Autodesk Fusion 360 part; units mm, degrees
(part 4 of 6)
  spline S1122 degree 3 poles (-50.344, 15.3773) (-50.4556, 15.307) (-50.5645, 15.241) (-50.6872, 15.1921) knots 0 0 0 0 1 1 1 1
  spline S1123 degree 3 poles (-50.6872, 15.1921) (-50.6691, 15.2109) (-50.651, 15.2297) (-50.6323, 15.2491) knots 0 0 0 0 1 1 1 1
  spline S1124 degree 3 poles (-50.6323, 15.2491) (-50.4501, 15.4534) (-50.3811, 15.6233) (-50.3221, 15.8884) knots 0 0 0 0 1 1 1 1
  spline S1125 degree 3 poles (-50.3221, 15.8884) (-50.1794, 16.4731) (-49.682, 16.8133) (-49.2179, 17.1446) knots 0 0 0 0 1 1 1 1
  spline S1126 degree 3 poles (-49.2179, 17.1446) (-49.0182, 17.2877) (-48.8217, 17.435) (-48.6251, 17.5823) knots 0 0 0 0 1 1 1 1
  spline S1127 degree 3 poles (-48.6251, 17.5823) (-48.5603, 17.6304) (-48.4948, 17.6776) (-48.4293, 17.7247) knots 0 0 0 0 1 1 1 1
  spline S1128 degree 3 poles (-48.4293, 17.7247) (-48.0216, 18.0274) (-47.557, 18.5172) (-47.4394, 19.0281) knots 0 0 0 0 1 1 1 1
  spline S1129 degree 3 poles (-47.4394, 19.0281) (-47.463, 19.2434) (-47.4932, 19.4392) (-47.6255, 19.6149) knots 0 0 0 0 1 1 1 1
  spline S1130 degree 3 poles (-47.6255, 19.6149) (-48.0279, 19.8024) (-48.4467, 19.7521) (-48.8536, 19.61) knots 0 0 0 0 1 1 1 1
  spline S1131 degree 3 poles (-48.8536, 19.61) (-49.2499, 19.4463) (-49.6121, 19.2138) (-49.9763, 18.9893) knots 0 0 0 0 1 1 1 1
  spline S1132 degree 3 poles (-49.9763, 18.9893) (-50.2765, 18.8143) (-50.6627, 18.7282) (-51.0047, 18.8097) knots 0 0 0 0 1 1 1 1
  spline S1133 degree 3 poles (-51.0047, 18.8097) (-51.0936, 18.8443) (-51.1659, 18.8904) (-51.2454, 18.943) knots 0 0 0 0 1 1 1 1
  spline S1134 degree 3 poles (-51.2454, 18.943) (-51.389, 19.034) (-51.4771, 19.0454) (-51.6426, 19.014) knots 0 0 0 0 1 1 1 1
  spline S1135 degree 3 poles (-51.6426, 19.014) (-51.7259, 18.9745) (-51.7259, 18.9745) (-51.8388, 18.8732) knots 0 0 0 0 1 1 1 1
  spline S1136 degree 3 poles (-51.8388, 18.8732) (-51.9741, 18.7595) (-52.1019, 18.7139) (-52.2735, 18.6677) knots 0 0 0 0 1 1 1 1
  spline S1137 degree 3 poles (-52.2735, 18.6677) (-52.331, 18.6516) (-52.3884, 18.6356) (-52.4459, 18.6195) knots 0 0 0 0 1 1 1 1
  spline S1138 degree 3 poles (-52.4459, 18.6195) (-52.4756, 18.6115) (-52.5054, 18.6034) (-52.536, 18.5951) knots 0 0 0 0 1 1 1 1
  spline S1139 degree 3 poles (-52.536, 18.5951) (-53.1106, 18.439) (-53.6573, 18.2525) (-54.198, 18.0016) knots 0 0 0 0 1 1 1 1
  spline S1140 degree 3 poles (-54.198, 18.0016) (-54.6047, 17.814) (-55.0066, 17.6569) (-55.4376, 17.5352) knots 0 0 0 0 1 1 1 1
  spline S1141 degree 3 poles (-55.4376, 17.5352) (-55.4604, 17.5687) (-55.4604, 17.5687) (-55.4836, 17.6029) knots 0 0 0 0 1 1 1 1
  spline S1142 degree 3 poles (-55.4836, 17.6029) (-55.6209, 17.7753) (-55.8226, 17.8559) (-56.0361, 17.884) knots 0 0 0 0 1 1 1 1
  spline S1143 degree 3 poles (-56.0361, 17.884) (-56.1445, 17.8761) (-56.2456, 17.8642) (-56.3522, 17.8463) knots 0 0 0 0 1 1 1 1
  spline S1144 degree 3 poles (-56.3522, 17.8463) (-56.3919, 17.8414) (-56.3919, 17.8414) (-56.4323, 17.8363) knots 0 0 0 0 1 1 1 1
  spline S1145 degree 3 poles (-56.4323, 17.8363) (-57.0096, 17.7406) (-57.5367, 17.3205) (-58.0104, 16.9992) knots 0 0 0 0 1 1 1 1
  spline S1146 degree 3 poles (-58.0104, 16.9992) (-58.3797, 16.7497) (-58.7477, 16.5551) (-59.1587, 16.3833) knots 0 0 0 0 1 1 1 1
  spline S1147 degree 3 poles (-59.1587, 16.3833) (-59.2277, 16.3521) (-59.2965, 16.3206) (-59.3651, 16.2885) knots 0 0 0 0 1 1 1 1
  spline S1148 degree 3 poles (-59.3651, 16.2885) (-59.3944, 16.275) (-59.4236, 16.2614) (-59.4537, 16.2474) knots 0 0 0 0 1 1 1 1
  spline S1149 degree 3 poles (-59.4537, 16.2474) (-59.5111, 16.2206) (-59.5686, 16.1938) (-59.626, 16.167) knots 0 0 0 0 1 1 1 1
  spline S1150 degree 3 poles (-59.626, 16.167) (-59.6549, 16.1536) (-59.6837, 16.1402) (-59.7135, 16.1264) knots 0 0 0 0 1 1 1 1
  spline S1151 degree 3 poles (-59.7135, 16.1264) (-59.7417, 16.1133) (-59.7699, 16.1002) (-59.7989, 16.0867) knots 0 0 0 0 1 1 1 1
  spline S1152 degree 3 poles (-59.7989, 16.0867) (-59.8853, 16.0485) (-59.9727, 16.015) (-60.0609, 15.9812) knots 0 0 0 0 1 1 1 1
  spline S1153 degree 3 poles (-60.0609, 15.9812) (-60.2413, 15.907) (-60.3774, 15.8013) (-60.5265, 15.6775) knots 0 0 0 0 1 1 1 1
  spline S1154 degree 3 poles (-60.5265, 15.6775) (-60.8228, 15.4401) (-61.1293, 15.22) (-61.4422, 15.0053) knots 0 0 0 0 1 1 1 1
  spline S1155 degree 3 poles (-61.4422, 15.0053) (-61.4931, 14.9704) (-61.544, 14.9352) (-61.5948, 14.9) knots 0 0 0 0 1 1 1 1
  spline S1156 degree 3 poles (-61.5948, 14.9) (-61.667, 14.85) (-61.7395, 14.8004) (-61.8121, 14.751) knots 0 0 0 0 1 1 1 1
  spline S1157 degree 3 poles (-61.8121, 14.751) (-61.8541, 14.7222) (-61.8962, 14.6934) (-61.9395, 14.6637) knots 0 0 0 0 1 1 1 1
  spline S1158 degree 3 poles (-61.9395, 14.6637) (-62.1493, 14.5407) (-62.3244, 14.4856) (-62.5654, 14.5176) knots 0 0 0 0 1 1 1 1
  spline S1159 degree 3 poles (-62.5654, 14.5176) (-63.3565, 14.5876) (-64.0549, 14.3462) (-64.6704, 13.8507) knots 0 0 0 0 1 1 1 1
  spline S1160 degree 3 poles (-64.6704, 13.8507) (-64.9868, 13.5794) (-65.2483, 13.2746) (-65.5102, 12.952) knots 0 0 0 0 1 1 1 1
  spline S1161 degree 3 poles (-65.5102, 12.952) (-65.5405, 12.9147) (-65.5405, 12.9147) (-65.5715, 12.8767) knots 0 0 0 0 1 1 1 1
  spline S1162 degree 3 poles (-65.5715, 12.8767) (-65.6101, 12.8292) (-65.6485, 12.7816) (-65.6867, 12.7337) knots 0 0 0 0 1 1 1 1
  spline S1163 degree 3 poles (-65.6867, 12.7337) (-66.0286, 12.3111) (-66.4249, 11.9667) (-66.8463, 11.6259) knots 0 0 0 0 1 1 1 1
  spline S1164 degree 3 poles (-66.8463, 11.6259) (-67.102, 11.4159) (-67.3243, 11.1965) (-67.5345, 10.941) knots 0 0 0 0 1 1 1 1
  spline S1165 degree 3 poles (-67.5345, 10.941) (-67.5595, 10.9112) (-67.5845, 10.8815) (-67.6103, 10.8508) knots 0 0 0 0 1 1 1 1
  spline S1166 degree 3 poles (-67.6103, 10.8508) (-68.0141, 10.3567) (-68.1173, 9.5556) (-68.0597, 8.9377) knots 0 0 0 0 1 1 1 1
  spline S1167 degree 3 poles (-68.0597, 8.9377) (-67.8934, 7.6051) (-67.2744, 6.568) (-66.5667, 5.4526) knots 0 0 0 0 1 1 1 1
  spline S1168 degree 3 poles (-66.5667, 5.4526) (-66.5415, 5.4125) (-66.5163, 5.3724) (-66.4904, 5.3311) knots 0 0 0 0 1 1 1 1
  spline S1169 degree 3 poles (-66.4904, 5.3311) (-66.4655, 5.2916) (-66.4405, 5.2522) (-66.4148, 5.2115) knots 0 0 0 0 1 1 1 1
  spline S1170 degree 3 poles (-66.4148, 5.2115) (-66.3924, 5.1759) (-66.37, 5.1403) (-66.3468, 5.1036) knots 0 0 0 0 1 1 1 1
  spline S1171 degree 3 poles (-66.3468, 5.1036) (-66.1436, 4.8029) (-65.891, 4.673) (-65.5627, 4.5317) knots 0 0 0 0 1 1 1 1
  spline S1172 degree 3 poles (-65.5627, 4.5317) (-65.4217, 4.4709) (-65.2852, 4.4033) (-65.1485, 4.3335) knots 0 0 0 0 1 1 1 1
  spline S1173 degree 3 poles (-65.1485, 4.3335) (-64.5048, 4.0056) (-63.893, 3.8018) (-63.1622, 3.8179) knots 0 0 0 0 1 1 1 1
  spline S1174 degree 3 poles (-63.1622, 3.8179) (-63.0974, 3.8188) (-63.0974, 3.8188) (-63.0313, 3.8198) knots 0 0 0 0 1 1 1 1
  spline S1175 degree 3 poles (-63.0313, 3.8198) (-62.9408, 3.8211) (-62.8502, 3.8227) (-62.7596, 3.8245) knots 0 0 0 0 1 1 1 1
  spline S1176 degree 3 poles (-62.7596, 3.8245) (-62.622, 3.8272) (-62.4844, 3.8293) (-62.3467, 3.8313) knots 0 0 0 0 1 1 1 1
  spline S1177 degree 3 poles (-62.3467, 3.8313) (-62.2582, 3.8327) (-62.1696, 3.8341) (-62.081, 3.8356) knots 0 0 0 0 1 1 1 1
  spline S1178 degree 3 poles (-62.081, 3.8356) (-62.0201, 3.8366) (-62.0201, 3.8366) (-61.958, 3.8376) knots 0 0 0 0 1 1 1 1
  spline S1179 degree 3 poles (-61.958, 3.8376) (-60.1229, 3.8743) (-58.2945, 4.4626) (-56.8097, 5.5496) knots 0 0 0 0 1 1 1 1
  spline S1180 degree 3 poles (-56.8097, 5.5496) (-56.6794, 5.6468) (-56.6794, 5.6468) (-56.5257, 5.6878) knots 0 0 0 0 1 1 1 1
  spline S1181 degree 3 poles (-56.5257, 5.6878) (-56.439, 5.6747) (-56.439, 5.6747) (-56.3829, 5.6059) knots 0 0 0 0 1 1 1 1
  spline S1182 degree 3 poles (-56.3829, 5.6059) (-56.2885, 5.4409) (-56.2394, 5.2593) (-56.1818, 5.0789) knots 0 0 0 0 1 1 1 1
  spline S1183 degree 3 poles (-56.1818, 5.0789) (-56.1663, 5.031) (-56.1509, 4.983) (-56.1349, 4.9336) knots 0 0 0 0 1 1 1 1
  spline S1184 degree 3 poles (-56.1349, 4.9336) (-55.9815, 4.4497) (-55.8516, 3.9594) (-55.7199, 3.4693) knots 0 0 0 0 1 1 1 1
  spline S1185 degree 3 poles (-55.7199, 3.4693) (-55.1814, 1.4664) (-54.5799, -0.5857) (-52.7021, -1.7273) knots 0 0 0 0 1 1 1 1
  spline S1186 degree 3 poles (-52.7021, -1.7273) (-52.1368, -2.0407) (-52.1368, -2.0407) (-51.9904, -2.0149) knots 0 0 0 0 1 1 1 1
  spline S1187 degree 3 poles (-51.9904, -2.0149) (-51.9906, -2.0524) (-51.9908, -2.0899) (-51.991, -2.1286) knots 0 0 0 0 1 1 1 1
  spline S1188 degree 3 poles (-51.991, -2.1286) (-51.9636, -2.8299) (-51.645, -3.4042) (-51.3097, -4.0015) knots 0 0 0 0 1 1 1 1
  spline S1189 degree 3 poles (-51.3097, -4.0015) (-51.3453, -4.0094) (-51.3453, -4.0094) (-51.3816, -4.0174) knots 0 0 0 0 1 1 1 1
  spline S1190 degree 3 poles (-51.3816, -4.0174) (-52.0739, -4.1867) (-52.7152, -4.5109) (-53.2315, -5.0035) knots 0 0 0 0 1 1 1 1
  spline S1191 degree 3 poles (-53.2315, -5.0035) (-53.3705, -5.1323) (-53.4674, -5.2003) (-53.6593, -5.2006) knots 0 0 0 0 1 1 1 1
  spline S1192 degree 3 poles (-53.6593, -5.2006) (-53.7599, -5.1657) (-53.8483, -5.129) (-53.9434, -5.0829) knots 0 0 0 0 1 1 1 1
  spline S1193 degree 3 poles (-53.9434, -5.0829) (-55.9004, -4.2074) (-58.0187, -5.0468) (-59.9027, -5.7123) knots 0 0 0 0 1 1 1 1
  spline S1194 degree 3 poles (-59.9027, -5.7123) (-60.2035, -5.8184) (-60.5051, -5.9214) (-60.8077, -6.0222) knots 0 0 0 0 1 1 1 1
  spline S1195 degree 3 poles (-60.8077, -6.0222) (-60.8482, -6.0358) (-60.8886, -6.0493) (-60.9303, -6.0633) knots 0 0 0 0 1 1 1 1
  spline S1196 degree 3 poles (-60.9303, -6.0633) (-61.0381, -6.099) (-61.1461, -6.1339) (-61.2544, -6.1681) knots 0 0 0 0 1 1 1 1
  spline S1197 degree 3 poles (-61.2544, -6.1681) (-61.2996, -6.1825) (-61.2996, -6.1825) (-61.3456, -6.1972) knots 0 0 0 0 1 1 1 1
  spline S1198 degree 3 poles (-61.3456, -6.1972) (-61.6363, -6.2846) (-61.934, -6.3369) (-62.2324, -6.3895) knots 0 0 0 0 1 1 1 1
  spline S1199 degree 3 poles (-62.2324, -6.3895) (-62.3222, -6.4054) (-62.4119, -6.422) (-62.5016, -6.4386) knots 0 0 0 0 1 1 1 1
  spline S1200 degree 3 poles (-62.5016, -6.4386) (-63.1944, -6.5706) (-63.1944, -6.5706) (-63.8495, -6.3701) knots 0 0 0 0 1 1 1 1
  spline S1201 degree 3 poles (-63.8495, -6.3701) (-63.8786, -6.3546) (-63.9077, -6.339) (-63.9377, -6.323) knots 0 0 0 0 1 1 1 1
  spline S1202 degree 3 poles (-63.9377, -6.323) (-63.9949, -6.2924) (-64.0519, -6.2614) (-64.1086, -6.2299) knots 0 0 0 0 1 1 1 1
  spline S1203 degree 3 poles (-64.1086, -6.2299) (-64.1998, -6.18) (-64.2933, -6.1357) (-64.3868, -6.0905) knots 0 0 0 0 1 1 1 1
  spline S1204 degree 3 poles (-64.3868, -6.0905) (-64.5845, -5.986) (-64.761, -5.8541) (-64.942, -5.7237) knots 0 0 0 0 1 1 1 1
  spline S1205 degree 3 poles (-64.942, -5.7237) (-65.255, -5.4989) (-65.5487, -5.3398) (-65.9234, -5.2384) knots 0 0 0 0 1 1 1 1
  spline S1206 degree 3 poles (-65.9234, -5.2384) (-66.0477, -5.198) (-66.1425, -5.1475) (-66.2555, -5.0827) knots 0 0 0 0 1 1 1 1
  spline S1207 degree 3 poles (-66.2555, -5.0827) (-67.2908, -4.5046) (-68.5469, -4.3059) (-69.7187, -4.3147) knots 0 0 0 0 1 1 1 1
  spline S1208 degree 3 poles (-69.7187, -4.3147) (-69.7712, -4.3147) (-69.8237, -4.3147) (-69.8778, -4.3147) knots 0 0 0 0 1 1 1 1
  spline S1209 degree 3 poles (-69.8778, -4.3147) (-70.2207, -4.3231) (-70.5539, -4.37) (-70.8918, -4.426) knots 0 0 0 0 1 1 1 1
  spline S1210 degree 3 poles (-70.8918, -4.426) (-70.9339, -4.4327) (-70.9759, -4.4394) (-71.0192, -4.4463) knots 0 0 0 0 1 1 1 1
  spline S1211 degree 3 poles (-71.0192, -4.4463) (-71.5269, -4.5363) (-71.9207, -4.7633) (-72.2275, -5.1851) knots 0 0 0 0 1 1 1 1
  spline S1212 degree 3 poles (-72.2275, -5.1851) (-72.3637, -5.399) (-72.4828, -5.6214) (-72.5986, -5.8468) knots 0 0 0 0 1 1 1 1
  spline S1213 degree 3 poles (-72.5986, -5.8468) (-72.6546, -5.9506) (-72.7163, -6.0487) (-72.7801, -6.1479) knots 0 0 0 0 1 1 1 1
  spline S1214 degree 3 poles (-72.7801, -6.1479) (-72.9035, -6.3449) (-72.9941, -6.549) (-73.0848, -6.7625) knots 0 0 0 0 1 1 1 1
  spline S1215 degree 3 poles (-73.0848, -6.7625) (-73.2634, -7.1723) (-73.4816, -7.563) (-73.7041, -7.9502) knots 0 0 0 0 1 1 1 1
  spline S1216 degree 3 poles (-73.7041, -7.9502) (-73.7179, -7.9743) (-73.7316, -7.9983) (-73.7458, -8.023) knots 0 0 0 0 1 1 1 1
  spline S1217 degree 3 poles (-73.7458, -8.023) (-73.9174, -8.3215) (-74.0931, -8.6166) (-74.2768, -8.9079) knots 0 0 0 0 1 1 1 1
  spline S1218 degree 3 poles (-74.2768, -8.9079) (-74.3558, -9.0336) (-74.4324, -9.1607) (-74.5089, -9.288) knots 0 0 0 0 1 1 1 1
  spline S1219 degree 3 poles (-74.5089, -9.288) (-74.5741, -9.3949) (-74.6411, -9.5007) (-74.708, -9.6066) knots 0 0 0 0 1 1 1 1
  spline S1220 degree 3 poles (-74.708, -9.6066) (-74.8384, -9.8136) (-74.9561, -10.0259) (-75.0703, -10.2421) knots 0 0 0 0 1 1 1 1
  spline S1221 degree 3 poles (-75.0703, -10.2421) (-75.143, -10.3569) (-75.2065, -10.4303) (-75.3186, -10.5068) knots 0 0 0 0 1 1 1 1
  spline S1222 degree 3 poles (-75.3186, -10.5068) (-75.4881, -10.5374) (-75.6201, -10.4209) (-75.755, -10.3308) knots 0 0 0 0 1 1 1 1
  spline S1223 degree 3 poles (-75.755, -10.3308) (-75.7812, -10.3136) (-75.8075, -10.2965) (-75.8345, -10.2788) knots 0 0 0 0 1 1 1 1
  spline S1224 degree 3 poles (-75.8345, -10.2788) (-76.0434, -10.1412) (-76.2473, -9.9967) (-76.4513, -9.852) knots 0 0 0 0 1 1 1 1
  spline S1225 degree 3 poles (-76.4513, -9.852) (-76.7266, -9.6571) (-77.0027, -9.4835) (-77.3026, -9.3283) knots 0 0 0 0 1 1 1 1
  spline S1226 degree 3 poles (-77.3026, -9.3283) (-77.3412, -9.3073) (-77.3798, -9.2863) (-77.4196, -9.2647) knots 0 0 0 0 1 1 1 1
  spline S1227 degree 3 poles (-77.4196, -9.2647) (-78.1033, -8.9074) (-78.9925, -8.6536) (-79.7502, -8.8776) knots 0 0 0 0 1 1 1 1
  spline S1228 degree 3 poles (-79.7502, -8.8776) (-79.9183, -8.9311) (-80.083, -8.9914) (-80.2475, -9.055) knots 0 0 0 0 1 1 1 1
  spline S1229 degree 3 poles (-80.2475, -9.055) (-80.2801, -9.067) (-80.3128, -9.0791) (-80.3464, -9.0915) knots 0 0 0 0 1 1 1 1
  spline S1230 degree 3 poles (-80.3464, -9.0915) (-80.6659, -9.2148) (-80.9042, -9.3674) (-81.0849, -9.6647) knots 0 0 0 0 1 1 1 1
  spline S1231 degree 3 poles (-81.0849, -9.6647) (-81.1051, -9.6964) (-81.1254, -9.7281) (-81.1462, -9.7608) knots 0 0 0 0 1 1 1 1
  spline S1232 degree 3 poles (-81.1462, -9.7608) (-81.231, -9.9376) (-81.2647, -10.1121) (-81.3, -10.3042) knots 0 0 0 0 1 1 1 1
  spline S1233 degree 3 poles (-81.3, -10.3042) (-81.3073, -10.3437) (-81.3147, -10.3831) (-81.3223, -10.4238) knots 0 0 0 0 1 1 1 1
  spline S1234 degree 3 poles (-81.3223, -10.4238) (-81.5295, -11.5933) (-81.5096, -12.9952) (-80.9381, -14.071) knots 0 0 0 0 1 1 1 1
  spline S1235 degree 3 poles (-80.9381, -14.071) (-80.8732, -14.1963) (-80.8303, -14.2822) (-80.8599, -14.4236) knots 0 0 0 0 1 1 1 1
  spline S1236 degree 3 poles (-80.8599, -14.4236) (-80.9019, -14.5264) (-80.9506, -14.6213) (-81.0044, -14.7184) knots 0 0 0 0 1 1 1 1
  spline S1237 degree 3 poles (-81.0044, -14.7184) (-81.0227, -14.7536) (-81.041, -14.7887) (-81.0598, -14.825) knots 0 0 0 0 1 1 1 1
  spline S1238 degree 3 poles (-81.0598, -14.825) (-81.2073, -15.1051) (-81.3656, -15.3796) (-81.5308, -15.6497) knots 0 0 0 0 1 1 1 1
  spline S1239 degree 3 poles (-81.5308, -15.6497) (-81.5519, -15.6844) (-81.5519, -15.6844) (-81.5734, -15.7199) knots 0 0 0 0 1 1 1 1
  spline S1240 degree 3 poles (-81.5734, -15.7199) (-81.6024, -15.7672) (-81.6322, -15.8141) (-81.6626, -15.8605) knots 0 0 0 0 1 1 1 1
  spline S1241 degree 3 poles (-81.6626, -15.8605) (-81.818, -16.1078) (-81.7716, -16.2778) (-81.6891, -16.5457) knots 0 0 0 0 1 1 1 1
  spline S1242 degree 3 poles (-80.843, -15.9266) (-80.8068, -15.8705) (-80.771, -15.8142) (-80.7353, -15.7577) knots 0 0 0 0 1 1 1 1
  spline S1243 degree 3 poles (-80.7353, -15.7577) (-80.7071, -15.7131) (-80.7071, -15.7131) (-80.6784, -15.6676) knots 0 0 0 0 1 1 1 1
  spline S1244 degree 3 poles (-80.6784, -15.6676) (-80.5785, -15.5008) (-80.4954, -15.3263) (-80.4118, -15.1509) knots 0 0 0 0 1 1 1 1
  spline S1245 degree 3 poles (-80.4118, -15.1509) (-80.3882, -15.1016) (-80.3882, -15.1016) (-80.364, -15.0514) knots 0 0 0 0 1 1 1 1
  spline S1246 degree 3 poles (-80.364, -15.0514) (-80.3179, -14.9544) (-80.2728, -14.8571) (-80.2278, -14.7596) knots 0 0 0 0 1 1 1 1
  spline S1247 degree 3 poles (-80.2278, -14.7596) (-80.2108, -14.7238) (-80.1938, -14.6879) (-80.1762, -14.651) knots 0 0 0 0 1 1 1 1
  spline S1248 degree 3 poles (-80.1762, -14.651) (-80.1598, -14.6154) (-80.1433, -14.5799) (-80.1264, -14.5433) knots 0 0 0 0 1 1 1 1
  spline S1249 degree 3 poles (-80.1264, -14.5433) (-80.1114, -14.5112) (-80.0963, -14.4791) (-80.0809, -14.446) knots 0 0 0 0 1 1 1 1
  spline S1250 degree 3 poles (-80.0809, -14.446) (-80.0301, -14.294) (-80.0815, -14.1798) (-80.1476, -14.0433) knots 0 0 0 0 1 1 1 1
  spline S1251 degree 3 poles (-80.1476, -14.0433) (-80.6954, -12.8464) (-80.8903, -11.5151) (-80.5312, -10.228) knots 0 0 0 0 1 1 1 1
  spline S1252 degree 3 poles (-80.5312, -10.228) (-80.4467, -10.0048) (-80.3701, -9.8918) (-80.1541, -9.7898) knots 0 0 0 0 1 1 1 1
  spline S1253 degree 3 poles (-80.1541, -9.7898) (-79.4267, -9.4766) (-78.8032, -9.5039) (-78.0723, -9.7688) knots 0 0 0 0 1 1 1 1
  spline S1254 degree 3 poles (-78.0723, -9.7688) (-77.8734, -9.8526) (-77.6883, -9.9555) (-77.5031, -10.0659) knots 0 0 0 0 1 1 1 1
  spline S1255 degree 3 poles (-77.5031, -10.0659) (-77.4672, -10.0871) (-77.4314, -10.1083) (-77.3944, -10.1301) knots 0 0 0 0 1 1 1 1
  spline S1256 degree 3 poles (-77.3944, -10.1301) (-77.1271, -10.2928) (-76.8721, -10.4714) (-76.6168, -10.6519) knots 0 0 0 0 1 1 1 1
  spline S1257 degree 3 poles (-76.6168, -10.6519) (-76.4456, -10.7725) (-76.2734, -10.8881) (-76.0921, -10.9932) knots 0 0 0 0 1 1 1 1
  spline S1258 degree 3 poles (-76.0921, -10.9932) (-76.0312, -11.0288) (-75.9713, -11.0661) (-75.9121, -11.1044) knots 0 0 0 0 1 1 1 1
  spline S1259 degree 3 poles (-75.9121, -11.1044) (-75.8797, -11.1252) (-75.8474, -11.1459) (-75.814, -11.1673) knots 0 0 0 0 1 1 1 1
  spline S1260 degree 3 poles (-75.814, -11.1673) (-75.7711, -11.1954) (-75.7711, -11.1954) (-75.7274, -11.224) knots 0 0 0 0 1 1 1 1
  spline S1261 degree 3 poles (-75.7274, -11.224) (-75.5278, -11.3181) (-75.2741, -11.2787) (-75.0713, -11.2067) knots 0 0 0 0 1 1 1 1
  spline S1262 degree 3 poles (-75.0713, -11.2067) (-74.7292, -11.0157) (-74.5238, -10.8159) (-74.3492, -10.464) knots 0 0 0 0 1 1 1 1
  spline S1263 degree 3 poles (-74.3492, -10.464) (-74.264, -10.2977) (-74.1651, -10.1443) (-74.0624, -9.9884) knots 0 0 0 0 1 1 1 1
  spline S1264 degree 3 poles (-74.0624, -9.9884) (-74.0257, -9.9323) (-73.9891, -9.8762) (-73.9525, -9.8201) knots 0 0 0 0 1 1 1 1
  spline S1265 degree 3 poles (-73.9525, -9.8201) (-73.9355, -9.794) (-73.9185, -9.768) (-73.9009, -9.7411) knots 0 0 0 0 1 1 1 1
  spline S1266 degree 3 poles (-73.9009, -9.7411) (-73.8072, -9.5965) (-73.7188, -9.4489) (-73.6312, -9.3005) knots 0 0 0 0 1 1 1 1
  spline S1267 degree 3 poles (-73.6312, -9.3005) (-73.6026, -9.2523) (-73.5739, -9.204) (-73.5452, -9.1558) knots 0 0 0 0 1 1 1 1
  spline S1268 degree 3 poles (-73.5452, -9.1558) (-73.4792, -9.0446) (-73.4135, -8.9333) (-73.3479, -8.8218) knots 0 0 0 0 1 1 1 1
  spline S1269 degree 3 poles (-73.3479, -8.8218) (-73.2869, -8.7183) (-73.2255, -8.615) (-73.1634, -8.5121) knots 0 0 0 0 1 1 1 1
  spline S1270 degree 3 poles (-73.1634, -8.5121) (-72.8339, -7.9621) (-72.5505, -7.3864) (-72.2794, -6.8058) knots 0 0 0 0 1 1 1 1
  spline S1271 degree 3 poles (-72.2794, -6.8058) (-72.1743, -6.5811) (-72.0542, -6.3717) (-71.9187, -6.1639) knots 0 0 0 0 1 1 1 1
  spline S1272 degree 3 poles (-71.9187, -6.1639) (-71.8471, -6.0501) (-71.7853, -5.9338) (-71.7236, -5.8145) knots 0 0 0 0 1 1 1 1
  spline S1273 degree 3 poles (-71.7236, -5.8145) (-71.5966, -5.5778) (-71.4479, -5.3681) (-71.2082, -5.2383) knots 0 0 0 0 1 1 1 1
  spline S1274 degree 3 poles (-71.2082, -5.2383) (-70.3477, -5.0083) (-69.4148, -4.9839) (-68.5406, -5.1397) knots 0 0 0 0 1 1 1 1
  spline S1275 degree 3 poles (-68.5406, -5.1397) (-68.4876, -5.1476) (-68.4346, -5.1555) (-68.38, -5.1636) knots 0 0 0 0 1 1 1 1
  spline S1276 degree 3 poles (-68.38, -5.1636) (-67.7323, -5.2648) (-67.0898, -5.4522) (-66.5208, -5.7808) knots 0 0 0 0 1 1 1 1
  spline S1277 degree 3 poles (-66.5208, -5.7808) (-66.3054, -5.9041) (-66.0916, -5.9751) (-65.8541, -6.0481) knots 0 0 0 0 1 1 1 1
  spline S1278 degree 3 poles (-65.8541, -6.0481) (-65.6176, -6.127) (-65.439, -6.2519) (-65.2495, -6.4104) knots 0 0 0 0 1 1 1 1
  spline S1279 degree 3 poles (-65.2495, -6.4104) (-64.9135, -6.6853) (-64.5171, -6.862) (-64.1258, -7.0436) knots 0 0 0 0 1 1 1 1
  spline S1280 degree 3 poles (-64.1258, -7.0436) (-64.0896, -7.0607) (-64.0533, -7.0777) (-64.016, -7.0953) knots 0 0 0 0 1 1 1 1
  spline S1281 degree 3 poles (-64.016, -7.0953) (-63.8126, -7.1878) (-63.6441, -7.2436) (-63.4178, -7.2518) knots 0 0 0 0 1 1 1 1
  spline S1282 degree 3 poles (-63.4178, -7.2518) (-63.3923, -7.2548) (-63.3668, -7.2577) (-63.3405, -7.2608) knots 0 0 0 0 1 1 1 1
  spline S1283 degree 3 poles (-63.3405, -7.2608) (-63.0389, -7.2899) (-62.7461, -7.2269) (-62.4507, -7.1724) knots 0 0 0 0 1 1 1 1
  spline S1284 degree 3 poles (-62.4507, -7.1724) (-62.3595, -7.1555) (-62.2682, -7.1393) (-62.1769, -7.1233) knots 0 0 0 0 1 1 1 1
  spline S1285 degree 3 poles (-62.1769, -7.1233) (-61.4499, -6.9935) (-60.7697, -6.7941) (-60.075, -6.5462) knots 0 0 0 0 1 1 1 1
  spline S1286 degree 3 poles (-60.075, -6.5462) (-59.9895, -6.516) (-59.904, -6.4858) (-59.8185, -6.4556) knots 0 0 0 0 1 1 1 1
  spline S1287 degree 3 poles (-59.8185, -6.4556) (-59.6525, -6.397) (-59.4865, -6.3383) (-59.3206, -6.2794) knots 0 0 0 0 1 1 1 1
  spline S1288 degree 3 poles (-59.3206, -6.2794) (-58.9237, -6.1386) (-58.5263, -5.9994) (-58.1273, -5.8646) knots 0 0 0 0 1 1 1 1
  spline S1289 degree 3 poles (-58.1273, -5.8646) (-58.099, -5.8548) (-58.0707, -5.845) (-58.0416, -5.8349) knots 0 0 0 0 1 1 1 1
  spline S1290 degree 3 poles (-58.0416, -5.8349) (-57.2581, -5.5668) (-56.3383, -5.3727) (-55.5083, -5.4466) knots 0 0 0 0 1 1 1 1
  spline S1291 degree 3 poles (-55.5083, -5.4466) (-55.4746, -5.4496) (-55.441, -5.4525) (-55.4063, -5.4555) knots 0 0 0 0 1 1 1 1
  spline S1292 degree 3 poles (-55.4063, -5.4555) (-54.9068, -5.5065) (-54.4283, -5.6469) (-53.9729, -5.8571) knots 0 0 0 0 1 1 1 1
  spline S1293 degree 3 poles (-53.9729, -5.8571) (-53.7028, -5.9614) (-53.4421, -5.9531) (-53.1716, -5.8582) knots 0 0 0 0 1 1 1 1
  spline S1294 degree 3 poles (-53.1716, -5.8582) (-52.9314, -5.7114) (-52.7176, -5.5362) (-52.5139, -5.342) knots 0 0 0 0 1 1 1 1
  spline S1295 degree 3 poles (-52.5139, -5.342) (-52.1859, -5.039) (-51.7321, -4.8925) (-51.3214, -4.735) knots 0 0 0 0 1 1 1 1
  spline S1296 degree 3 poles (-51.3214, -4.735) (-51.2295, -4.6997) (-51.1378, -4.6639) (-51.0462, -4.6281) knots 0 0 0 0 1 1 1 1
  spline S1297 degree 3 poles (-51.0462, -4.6281) (-50.9872, -4.6052) (-50.9283, -4.5824) (-50.8694, -4.5596) knots 0 0 0 0 1 1 1 1
  spline S1298 degree 3 poles (-50.8694, -4.5596) (-50.8422, -4.549) (-50.8151, -4.5384) (-50.7871, -4.5275) knots 0 0 0 0 1 1 1 1
  spline S1299 degree 3 poles (-50.7871, -4.5275) (-50.6485, -4.4746) (-50.5167, -4.4335) (-50.3695, -4.414) knots 0 0 0 0 1 1 1 1
  spline S1300 degree 3 poles (-50.3695, -4.414) (-50.4824, -4.0391) (-50.6371, -3.7061) (-50.8258, -3.3637) knots 0 0 0 0 1 1 1 1
  spline S1301 degree 3 poles (-50.8258, -3.3637) (-50.8757, -3.2724) (-50.9254, -3.1811) (-50.975, -3.0896) knots 0 0 0 0 1 1 1 1
  spline S1302 degree 3 poles (-50.975, -3.0896) (-50.9968, -3.0499) (-51.0186, -3.0102) (-51.0411, -2.9693) knots 0 0 0 0 1 1 1 1
  spline S1303 degree 3 poles (-51.0411, -2.9693) (-51.1903, -2.664) (-51.2838, -2.3242) (-51.2366, -1.9852) knots 0 0 0 0 1 1 1 1
  spline S1304 degree 3 poles (-51.2366, -1.9852) (-51.2267, -1.8226) (-51.2649, -1.7413) (-51.3643, -1.6127) knots 0 0 0 0 1 1 1 1
  spline S1305 degree 3 poles (-51.3643, -1.6127) (-51.5348, -1.4371) (-51.7203, -1.3576) (-51.9451, -1.268) knots 0 0 0 0 1 1 1 1
  spline S1306 degree 3 poles (-51.9451, -1.268) (-52.877, -0.8772) (-53.5414, -0.1547) (-54.0025, 0.7284) knots 0 0 0 0 1 1 1 1
  spline S1307 degree 3 poles (-54.0025, 0.7284) (-54.0163, 0.7548) (-54.0301, 0.7812) (-54.0443, 0.8084) knots 0 0 0 0 1 1 1 1
  spline S1308 degree 3 poles (-54.0443, 0.8084) (-54.2299, 1.1713) (-54.3741, 1.5452) (-54.5022, 1.9317) knots 0 0 0 0 1 1 1 1
  spline S1309 degree 3 poles (-54.5022, 1.9317) (-54.5173, 1.9773) (-54.5325, 2.0228) (-54.548, 2.0697) knots 0 0 0 0 1 1 1 1
  spline S1310 degree 3 poles (-54.548, 2.0697) (-54.7227, 2.6035) (-54.8713, 3.1443) (-55.0197, 3.6858) knots 0 0 0 0 1 1 1 1
  spline S1311 degree 3 poles (-55.0197, 3.6858) (-55.1844, 4.2866) (-55.3525, 4.8853) (-55.5448, 5.478) knots 0 0 0 0 1 1 1 1
  spline S1312 degree 3 poles (-55.5448, 5.478) (-55.5596, 5.524) (-55.5744, 5.57) (-55.5897, 5.6174) knots 0 0 0 0 1 1 1 1
  spline S1313 degree 3 poles (-55.5897, 5.6174) (-55.6108, 5.6814) (-55.6108, 5.6814) (-55.6323, 5.7466) knots 0 0 0 0 1 1 1 1
  spline S1314 degree 3 poles (-55.6323, 5.7466) (-55.6446, 5.7839) (-55.6569, 5.8212) (-55.6695, 5.8597) knots 0 0 0 0 1 1 1 1
  spline S1315 degree 3 poles (-55.6695, 5.8597) (-55.7361, 6.0276) (-55.809, 6.152) (-55.9619, 6.2503) knots 0 0 0 0 1 1 1 1
  spline S1316 degree 3 poles (-55.9619, 6.2503) (-55.9879, 6.267) (-56.0138, 6.2837) (-56.0406, 6.301) knots 0 0 0 0 1 1 1 1
  spline S1317 degree 3 poles (-56.0406, 6.301) (-56.0676, 6.3178) (-56.0945, 6.3346) (-56.1223, 6.3519) knots 0 0 0 0 1 1 1 1
  spline S1318 degree 3 poles (-56.1223, 6.3519) (-56.1621, 6.3779) (-56.1621, 6.3779) (-56.2028, 6.4044) knots 0 0 0 0 1 1 1 1
  spline S1319 degree 3 poles (-56.2028, 6.4044) (-56.3492, 6.4973) (-56.469, 6.5672) (-56.6457, 6.5823) knots 0 0 0 0 1 1 1 1
  spline S1320 degree 3 poles (-56.6457, 6.5823) (-56.7423, 6.5337) (-56.7423, 6.5337) (-56.8407, 6.4577) knots 0 0 0 0 1 1 1 1
  spline S1321 degree 3 poles (-56.8407, 6.4577) (-56.8775, 6.4301) (-56.9143, 6.4024) (-56.9523, 6.3739) knots 0 0 0 0 1 1 1 1
  spline S1322 degree 3 poles (-56.9523, 6.3739) (-56.9913, 6.3438) (-57.0303, 6.3138) (-57.0705, 6.2828) knots 0 0 0 0 1 1 1 1
  spline S1323 degree 3 poles (-57.0705, 6.2828) (-57.4699, 5.9861) (-57.871, 5.7285) (-58.3142, 5.5032) knots 0 0 0 0 1 1 1 1
  spline S1324 degree 3 poles (-58.3142, 5.5032) (-58.3475, 5.4862) (-58.3807, 5.4692) (-58.4149, 5.4516) knots 0 0 0 0 1 1 1 1
  spline S1325 degree 3 poles (-58.4149, 5.4516) (-59.858, 4.7202) (-61.3405, 4.5436) (-62.939, 4.5496) knots 0 0 0 0 1 1 1 1
  spline S1326 degree 3 poles (-62.939, 4.5496) (-63.0584, 4.5495) (-63.1777, 4.5469) (-63.297, 4.5446) knots 0 0 0 0 1 1 1 1
  spline S1327 degree 3 poles (-63.297, 4.5446) (-63.7747, 4.5401) (-64.1846, 4.6787) (-64.6085, 4.8891) knots 0 0 0 0 1 1 1 1
  spline S1328 degree 3 poles (-64.6085, 4.8891) (-64.6377, 4.9035) (-64.6669, 4.918) (-64.6969, 4.9329) knots 0 0 0 0 1 1 1 1
  spline S1329 degree 3 poles (-64.6969, 4.9329) (-64.8806, 5.0244) (-65.0638, 5.1169) (-65.2456, 5.212) knots 0 0 0 0 1 1 1 1
  spline S1330 degree 3 poles (-65.2456, 5.212) (-65.3066, 5.2428) (-65.3685, 5.272) (-65.431, 5.2997) knots 0 0 0 0 1 1 1 1
  spline S1331 degree 3 poles (-65.431, 5.2997) (-65.65, 5.3995) (-65.7528, 5.4853) (-65.8677, 5.7049) knots 0 0 0 0 1 1 1 1
  spline S1332 degree 3 poles (-65.8677, 5.7049) (-65.897, 5.7588) (-65.9264, 5.8127) (-65.9559, 5.8665) knots 0 0 0 0 1 1 1 1
  spline S1333 degree 3 poles (-65.9559, 5.8665) (-65.9711, 5.8948) (-65.9863, 5.923) (-66.002, 5.9522) knots 0 0 0 0 1 1 1 1
  spline S1334 degree 3 poles (-66.002, 5.9522) (-66.0685, 6.0715) (-66.1416, 6.1862) (-66.215, 6.3014) knots 0 0 0 0 1 1 1 1
  spline S1335 degree 3 poles (-66.215, 6.3014) (-66.4131, 6.6128) (-66.5985, 6.9302) (-66.7759, 7.2538) knots 0 0 0 0 1 1 1 1
  spline S1336 degree 3 poles (-66.7759, 7.2538) (-66.7961, 7.2902) (-66.8163, 7.3265) (-66.8371, 7.364) knots 0 0 0 0 1 1 1 1
  spline S1337 degree 3 poles (-66.8371, 7.364) (-67.2901, 8.2014) (-67.4687, 9.1631) (-67.2022, 10.0832) knots 0 0 0 0 1 1 1 1
  spline S1338 degree 3 poles (-67.2022, 10.0832) (-66.9956, 10.6318) (-66.4475, 10.9921) (-66.0162, 11.3556) knots 0 0 0 0 1 1 1 1
  spline S1339 degree 3 poles (-66.0162, 11.3556) (-65.6401, 11.674) (-65.3148, 12.0154) (-65.0181, 12.4096) knots 0 0 0 0 1 1 1 1
  spline S1340 degree 3 poles (-65.0181, 12.4096) (-64.5632, 13.0027) (-64.0203, 13.6014) (-63.2562, 13.7349) knots 0 0 0 0 1 1 1 1
  spline S1341 degree 3 poles (-63.2562, 13.7349) (-63.2209, 13.7411) (-63.1857, 13.7474) (-63.1493, 13.7538) knots 0 0 0 0 1 1 1 1
  spline S1342 degree 3 poles (-63.1493, 13.7538) (-62.8338, 13.804) (-62.5593, 13.7819) (-62.2437, 13.7327) knots 0 0 0 0 1 1 1 1
  spline S1343 degree 3 poles (-62.2437, 13.7327) (-62.0559, 13.7096) (-61.9695, 13.7559) (-61.8157, 13.8629) knots 0 0 0 0 1 1 1 1
  spline S1344 degree 3 poles (-61.8157, 13.8629) (-61.773, 13.8923) (-61.7302, 13.9216) (-61.6862, 13.9519) knots 0 0 0 0 1 1 1 1
  spline S1345 degree 3 poles (-61.6862, 13.9519) (-61.6402, 13.9842) (-61.5942, 14.0166) (-61.5482, 14.049) knots 0 0 0 0 1 1 1 1
  spline S1346 degree 3 poles (-61.5482, 14.049) (-61.5008, 14.0818) (-61.4533, 14.1147) (-61.4059, 14.1475) knots 0 0 0 0 1 1 1 1
  spline S1347 degree 3 poles (-61.4059, 14.1475) (-61.3079, 14.2152) (-61.2102, 14.2833) (-61.1126, 14.3515) knots 0 0 0 0 1 1 1 1
  spline S1348 degree 3 poles (-61.1126, 14.3515) (-60.972, 14.4498) (-60.8308, 14.5472) (-60.6894, 14.6443) knots 0 0 0 0 1 1 1 1
  spline S1349 degree 3 poles (-60.6894, 14.6443) (-60.6037, 14.7033) (-60.518, 14.7624) (-60.4323, 14.8214) knots 0 0 0 0 1 1 1 1
  spline S1350 degree 3 poles (-60.4323, 14.8214) (-60.3924, 14.849) (-60.3524, 14.8765) (-60.3113, 14.9049) knots 0 0 0 0 1 1 1 1
  spline S1351 degree 3 poles (-60.3113, 14.9049) (-60.2742, 14.9306) (-60.237, 14.9564) (-60.1988, 14.983) knots 0 0 0 0 1 1 1 1
  spline S1352 degree 3 poles (-60.1988, 14.983) (-60.1664, 15.0054) (-60.1341, 15.0278) (-60.1008, 15.0509) knots 0 0 0 0 1 1 1 1
  spline S1353 degree 3 poles (-60.1008, 15.0509) (-60.0096, 15.118) (-60.0096, 15.118) (-59.9245, 15.1963) knots 0 0 0 0 1 1 1 1
  spline S1354 degree 3 poles (-59.9245, 15.1963) (-59.8127, 15.2881) (-59.7018, 15.3405) (-59.5698, 15.3995) knots 0 0 0 0 1 1 1 1
  spline S1355 degree 3 poles (-59.5698, 15.3995) (-59.5324, 15.4164) (-59.5324, 15.4164) (-59.4942, 15.4337) knots 0 0 0 0 1 1 1 1
  spline S1356 degree 3 poles (-59.4942, 15.4337) (-59.4147, 15.4695) (-59.335, 15.5048) (-59.2553, 15.5402) knots 0 0 0 0 1 1 1 1
  spline S1357 degree 3 poles (-59.2553, 15.5402) (-59.2029, 15.5637) (-59.1505, 15.5872) (-59.0981, 15.6108) knots 0 0 0 0 1 1 1 1
  spline S1358 degree 3 poles (-59.0981, 15.6108) (-59.0464, 15.634) (-58.9947, 15.6572) (-58.943, 15.6804) knots 0 0 0 0 1 1 1 1
  spline S1359 degree 3 poles (-58.943, 15.6804) (-58.9173, 15.692) (-58.8916, 15.7035) (-58.8652, 15.7154) knots 0 0 0 0 1 1 1 1
  spline S1360 degree 3 poles (-58.8652, 15.7154) (-58.7527, 15.7657) (-58.64, 15.8151) (-58.5259, 15.8619) knots 0 0 0 0 1 1 1 1
  spline S1361 degree 3 poles (-58.5259, 15.8619) (-58.1822, 16.0049) (-57.8839, 16.2055) (-57.576, 16.412) knots 0 0 0 0 1 1 1 1
  spline S1362 degree 3 poles (-57.576, 16.412) (-56.8571, 16.9044) (-56.8571, 16.9044) (-56.0292, 17.1417) knots 0 0 0 0 1 1 1 1
  spline S1363 degree 3 poles (-56.0292, 17.1417) (-55.9382, 16.9737) (-55.9382, 16.9737) (-55.8454, 16.8023) knots 0 0 0 0 1 1 1 1
  spline S1364 degree 3 poles (-55.8454, 16.8023) (-55.0454, 16.7899) (-54.3208, 17.1105) (-53.6127, 17.449) knots 0 0 0 0 1 1 1 1
  spline S1365 degree 3 poles (-53.6127, 17.449) (-53.0429, 17.7197) (-52.4341, 17.8812) (-51.8254, 18.0386) knots 0 0 0 0 1 1 1 1
  spline S1366 degree 3 poles (-51.8254, 18.0386) (-51.7351, 18.0637) (-51.6477, 18.0933) (-51.5592, 18.1241) knots 0 0 0 0 1 1 1 1
  spline S1367 degree 3 poles (-51.5592, 18.1241) (-51.4253, 18.1713) (-51.4253, 18.1713) (-51.3221, 18.1385) knots 0 0 0 0 1 1 1 1
  spline S1368 degree 3 poles (-51.3221, 18.1385) (-51.2854, 18.1161) (-51.2854, 18.1161) (-51.2478, 18.0932) knots 0 0 0 0 1 1 1 1
  spline S1369 degree 3 poles (-51.2478, 18.0932) (-51.0088, 17.9531) (-50.8091, 18.0133) (-50.5474, 18.0592) knots 0 0 0 0 1 1 1 1
  spline S1370 degree 3 poles (-50.5474, 18.0592) (-50.5088, 18.0655) (-50.4702, 18.0718) (-50.4305, 18.0783) knots 0 0 0 0 1 1 1 1
  spline S1371 degree 3 poles (-50.4305, 18.0783) (-49.92, 18.1672) (-49.5286, 18.4106) (-49.0868, 18.6738) knots 0 0 0 0 1 1 1 1
  spline S1372 degree 3 poles (-49.0868, 18.6738) (-48.8304, 18.8232) (-48.5939, 18.9404) (-48.3019, 18.9999) knots 0 0 0 0 1 1 1 1
  spline S1373 degree 3 poles (-48.3019, 18.9999) (-48.451, 18.4355) (-49.259, 18.0164) (-49.7138, 17.695) knots 0 0 0 0 1 1 1 1
  spline S1374 degree 3 poles (-49.7138, 17.695) (-49.9996, 17.4927) (-50.2749, 17.2939) (-50.5173, 17.0396) knots 0 0 0 0 1 1 1 1
  spline S1375 degree 3 poles (-50.5173, 17.0396) (-50.5506, 17.0057) (-50.5506, 17.0057) (-50.5845, 16.9711) knots 0 0 0 0 1 1 1 1
  spline S1376 degree 3 poles (-50.5845, 16.9711) (-50.8231, 16.7068) (-50.9749, 16.3705) (-51.0537, 16.0259) knots 0 0 0 0 1 1 1 1
  spline S1377 degree 3 poles (-51.0537, 16.0259) (-51.1748, 15.5904) (-51.6679, 15.332) (-52.0375, 15.1193) knots 0 0 0 0 1 1 1 1
  spline S1378 degree 3 poles (-52.0375, 15.1193) (-52.5453, 14.8328) (-53.0658, 14.6059) (-53.6152, 14.4114) knots 0 0 0 0 1 1 1 1
  spline S1379 degree 3 poles (-53.6152, 14.4114) (-53.6575, 14.3964) (-53.6998, 14.3813) (-53.7433, 14.3659) knots 0 0 0 0 1 1 1 1
  spline S1380 degree 3 poles (-53.7433, 14.3659) (-53.7809, 14.3529) (-53.8184, 14.3399) (-53.857, 14.3265) knots 0 0 0 0 1 1 1 1
  spline S1381 degree 3 poles (-53.857, 14.3265) (-53.9531, 14.2865) (-54.0199, 14.2398) (-54.102, 14.1769) knots 0 0 0 0 1 1 1 1
  spline S1382 degree 3 poles (-54.102, 14.1769) (-54.4041, 14.0289) (-54.7342, 13.9604) (-55.0598, 13.8841) knots 0 0 0 0 1 1 1 1
  spline S1383 degree 3 poles (-55.0598, 13.8841) (-55.8147, 13.7071) (-56.4359, 13.4538) (-57.0158, 12.9274) knots 0 0 0 0 1 1 1 1
  spline S1384 degree 3 poles (-57.0158, 12.9274) (-57.7387, 12.2741) (-58.5573, 11.7907) (-59.4105, 11.3253) knots 0 0 0 0 1 1 1 1
  spline S1385 degree 3 poles (-59.4105, 11.3253) (-59.4665, 11.2945) (-59.4665, 11.2945) (-59.5236, 11.2631) knots 0 0 0 0 1 1 1 1
  spline S1386 degree 3 poles (-59.5236, 11.2631) (-59.6859, 11.1754) (-59.8444, 11.0942) (-60.0186, 11.033) knots 0 0 0 0 1 1 1 1
  spline S1387 degree 3 poles (-60.0186, 11.033) (-60.1637, 10.9816) (-60.2887, 10.9308) (-60.4108, 10.8339) knots 0 0 0 0 1 1 1 1
  spline S1388 degree 3 poles (-60.4108, 10.8339) (-60.5041, 10.624) (-60.5081, 10.4231) (-60.5051, 10.1977) knots 0 0 0 0 1 1 1 1
  spline S1389 degree 3 poles (-60.5051, 10.1977) (-60.5047, 10.1415) (-60.5047, 10.1415) (-60.5043, 10.0841) knots 0 0 0 0 1 1 1 1
  spline S1390 degree 3 poles (-60.5043, 10.0841) (-60.5013, 9.8341) (-60.4917, 9.5848) (-60.477, 9.3352) knots 0 0 0 0 1 1 1 1
  spline S1391 degree 3 poles (-60.477, 9.3352) (-60.4435, 9.331) (-60.41, 9.3268) (-60.3754, 9.3225) knots 0 0 0 0 1 1 1 1
  spline S1392 degree 3 poles (-60.3754, 9.3225) (-60.1845, 9.2913) (-59.9989, 9.2457) (-59.8112, 9.199) knots 0 0 0 0 1 1 1 1
  spline S1393 degree 3 poles (-59.8112, 9.199) (-59.7717, 9.1892) (-59.7322, 9.1795) (-59.6915, 9.1694) knots 0 0 0 0 1 1 1 1
  spline S1394 degree 3 poles (-59.6915, 9.1694) (-59.6079, 9.1488) (-59.5244, 9.1281) (-59.4409, 9.1074) knots 0 0 0 0 1 1 1 1
  spline S1395 degree 3 poles (-59.4409, 9.1074) (-59.3149, 9.0761) (-59.1888, 9.045) (-59.0627, 9.0139) knots 0 0 0 0 1 1 1 1
  spline S1396 degree 3 poles (-59.0627, 9.0139) (-58.9811, 8.9937) (-58.8995, 8.9735) (-58.8179, 8.9533) knots 0 0 0 0 1 1 1 1
  spline S1397 degree 3 poles (-58.8179, 8.9533) (-58.7781, 8.9435) (-58.7382, 8.9337) (-58.6972, 8.9235) knots 0 0 0 0 1 1 1 1
  spline S1398 degree 3 poles (-58.6972, 8.9235) (-58.5295, 8.8819) (-58.3622, 8.8399) (-58.196, 8.7927) knots 0 0 0 0 1 1 1 1
  spline S1399 degree 3 poles (-58.196, 8.7927) (-57.9145, 8.7132) (-57.6638, 8.6709) (-57.3713, 8.6772) knots 0 0 0 0 1 1 1 1
  spline S1400 degree 3 poles (-57.3713, 8.6772) (-57.2965, 8.6775) (-57.2216, 8.6778) (-57.1467, 8.6781) knots 0 0 0 0 1 1 1 1
  spline S1401 degree 3 poles (-57.1467, 8.6781) (-57.1106, 8.6784) (-57.0744, 8.6788) (-57.0372, 8.6791) knots 0 0 0 0 1 1 1 1
  spline S1402 degree 3 poles (-57.0372, 8.6791) (-56.8873, 8.6798) (-56.7378, 8.6753) (-56.588, 8.6707) knots 0 0 0 0 1 1 1 1
  spline S1403 degree 3 poles (-56.588, 8.6707) (-56.3843, 8.6662) (-56.186, 8.663) (-55.9832, 8.6818) knots 0 0 0 0 1 1 1 1
  spline S1404 degree 3 poles (-55.9832, 8.6818) (-55.9452, 8.6849) (-55.9072, 8.688) (-55.868, 8.6912) knots 0 0 0 0 1 1 1 1
  spline S1405 degree 3 poles (-55.868, 8.6912) (-55.6068, 8.7225) (-55.435, 8.7756) (-55.2554, 8.9722) knots 0 0 0 0 1 1 1 1
  spline S1406 degree 3 poles (-55.2554, 8.9722) (-55.082, 9.2122) (-54.9641, 9.4843) (-54.8486, 9.7556) knots 0 0 0 0 1 1 1 1
  spline S1407 degree 3 poles (-54.8486, 9.7556) (-54.6473, 10.2122) (-54.368, 10.6017) (-54.0767, 11.0056) knots 0 0 0 0 1 1 1 1
  spline S1408 degree 3 poles (-54.0767, 11.0056) (-53.955, 11.175) (-53.8421, 11.3468) (-53.7366, 11.5268) knots 0 0 0 0 1 1 1 1
  spline S1409 degree 3 poles (-53.7366, 11.5268) (-53.5458, 11.8505) (-53.2992, 12.1208) (-53.0467, 12.3968) knots 0 0 0 0 1 1 1 1
  spline S1410 degree 3 poles (-53.0467, 12.3968) (-52.9714, 12.4803) (-52.8977, 12.5649) (-52.824, 12.6498) knots 0 0 0 0 1 1 1 1
  spline S1411 degree 3 poles (-52.824, 12.6498) (-52.7848, 12.6945) (-52.7848, 12.6945) (-52.7447, 12.7402) knots 0 0 0 0 1 1 1 1
  spline S1412 degree 3 poles (-52.7447, 12.7402) (-52.6945, 12.7974) (-52.6447, 12.8549) (-52.5953, 12.9128) knots 0 0 0 0 1 1 1 1
  spline S1413 degree 3 poles (-52.5953, 12.9128) (-52.1805, 13.3812) (-51.6121, 13.6985) (-51.0893, 14.0318) knots 0 0 0 0 1 1 1 1
  spline S1414 degree 3 poles (-51.0893, 14.0318) (-51.0546, 14.0539) (-51.0199, 14.0761) (-50.9842, 14.0989) knots 0 0 0 0 1 1 1 1
  spline S1415 degree 3 poles (-50.9842, 14.0989) (-50.7388, 14.2558) (-50.4928, 14.4119) (-50.2467, 14.5676) knots 0 0 0 0 1 1 1 1
  spline S1416 degree 3 poles (-50.2467, 14.5676) (-50.2154, 14.5874) (-50.1842, 14.6071) (-50.1521, 14.6275) knots 0 0 0 0 1 1 1 1
  spline S1417 degree 3 poles (-50.1521, 14.6275) (-49.9826, 14.7347) (-49.8128, 14.8414) (-49.6425, 14.9471) knots 0 0 0 0 1 1 1 1
  spline S1418 degree 3 poles (-49.6425, 14.9471) (-49.5922, 14.9784) (-49.542, 15.0098) (-49.4918, 15.0413) knots 0 0 0 0 1 1 1 1
  spline S1419 degree 3 poles (-49.4918, 15.0413) (-49.0249, 15.3346) (-48.5604, 15.5499) (-48.0142, 15.6402) knots 0 0 0 0 1 1 1 1
  spline S1420 degree 3 poles (-48.0142, 15.6402) (-47.973, 15.6472) (-47.9318, 15.6541) (-47.8894, 15.6613) knots 0 0 0 0 1 1 1 1
  spline S1421 degree 3 poles (-47.8894, 15.6613) (-47.001, 15.7986) (-46.1205, 15.6398) (-45.2507, 15.4556) knots 0 0 0 0 1 1 1 1
  spline S1422 degree 3 poles (-45.2507, 15.4556) (-45.028, 15.4094) (-44.8161, 15.3764) (-44.589, 15.3664) knots 0 0 0 0 1 1 1 1
  spline S1423 degree 3 poles (-44.589, 15.3664) (-44.2414, 15.3451) (-43.9191, 15.2407) (-43.586, 15.1437) knots 0 0 0 0 1 1 1 1
  spline S1424 degree 3 poles (-43.586, 15.1437) (-43.3203, 15.0665) (-43.0561, 14.9936) (-42.7843, 14.9411) knots 0 0 0 0 1 1 1 1
  spline S1425 degree 3 poles (-42.7843, 14.9411) (-42.7329, 14.9311) (-42.6815, 14.9212) (-42.6286, 14.9109) knots 0 0 0 0 1 1 1 1
  spline S1426 degree 3 poles (-42.6286, 14.9109) (-42.314, 14.8872) (-42.0076, 15.1348) (-41.7781, 15.3317) knots 0 0 0 0 1 1 1 1
  spline S1427 degree 3 poles (-41.7781, 15.3317) (-41.4783, 15.6357) (-41.3069, 16.0072) (-41.1413, 16.3942) knots 0 0 0 0 1 1 1 1
  spline S1428 degree 3 poles (-41.1413, 16.3942) (-40.8962, 16.9627) (-40.5451, 17.4672) (-40.2043, 17.9814) knots 0 0 0 0 1 1 1 1
  spline S1429 degree 3 poles (-40.2043, 17.9814) (-39.9955, 18.2972) (-39.8061, 18.6156) (-39.6344, 18.9531) knots 0 0 0 0 1 1 1 1
  spline S1430 degree 3 poles (-39.6344, 18.9531) (-39.1983, 19.8061) (-38.6142, 20.6475) (-37.7209, 21.0722) knots 0 0 0 0 1 1 1 1
  spline S1431 degree 3 poles (-37.7209, 21.0722) (-37.437, 21.1572) (-37.1354, 21.243) (-36.8568, 21.1058) knots 0 0 0 0 1 1 1 1
  spline S1432 degree 3 poles (-36.8568, 21.1058) (-36.7593, 21.0426) (-36.7593, 21.0426) (-36.67, 20.9683) knots 0 0 0 0 1 1 1 1
  spline S1433 degree 3 poles (-36.67, 20.9683) (-36.6413, 20.9458) (-36.6126, 20.9233) (-36.5831, 20.9001) knots 0 0 0 0 1 1 1 1
  spline S1434 degree 3 poles (-36.5831, 20.9001) (-36.1762, 20.5359) (-35.9053, 20.0084) (-35.6632, 19.5257) knots 0 0 0 0 1 1 1 1
  spline S1435 degree 3 poles (-35.6632, 19.5257) (-35.4481, 19.0988) (-35.1834, 18.7125) (-34.8965, 18.3313) knots 0 0 0 0 1 1 1 1
  spline S1436 degree 3 poles (-34.8965, 18.3313) (-34.2054, 17.4119) (-33.597, 16.4486) (-33.0134, 15.4583) knots 0 0 0 0 1 1 1 1
  spline S1437 degree 3 poles (-33.0134, 15.4583) (-32.8231, 15.5624) (-32.6734, 15.7072) (-32.5151, 15.8534) knots 0 0 0 0 1 1 1 1
  spline S1438 degree 3 poles (-32.5151, 15.8534) (-32.4857, 15.8804) (-32.4562, 15.9074) (-32.4259, 15.9352) knots 0 0 0 0 1 1 1 1
  spline S1439 degree 3 poles (-32.4259, 15.9352) (-32.334, 16.0195) (-32.2424, 16.104) (-32.1509, 16.1887) knots 0 0 0 0 1 1 1 1
  spline S1440 degree 3 poles (-32.1509, 16.1887) (-32.1216, 16.2158) (-32.0923, 16.2428) (-32.0621, 16.2707) knots 0 0 0 0 1 1 1 1
  spline S1441 degree 3 poles (-32.0621, 16.2707) (-31.6307, 16.67) (-31.6307, 16.67) (-31.4415, 16.8508) knots 0 0 0 0 1 1 1 1
  spline S1442 degree 3 poles (-31.4415, 16.8508) (-31.245, 16.906) (-31.0372, 16.9343) (-30.8335, 16.9167) knots 0 0 0 0 1 1 1 1
  spline S1443 degree 3 poles (-30.8335, 16.9167) (-30.8289, 16.9439) (-30.8243, 16.9711) (-30.8196, 16.9992) knots 0 0 0 0 1 1 1 1
  spline S1444 degree 3 poles (-30.8196, 16.9992) (-30.79, 17.0978) (-30.79, 17.0978) (-30.6974, 17.1378) knots 0 0 0 0 1 1 1 1
  spline S1445 degree 3 poles (-30.6974, 17.1378) (-30.3269, 17.235) (-29.8658, 16.9264) (-29.5482, 16.7457) knots 0 0 0 0 1 1 1 1
  spline S1446 degree 3 poles (-29.5482, 16.7457) (-29.3761, 16.6448) (-29.2084, 16.5371) (-29.0414, 16.428) knots 0 0 0 0 1 1 1 1
  spline S1447 degree 3 poles (-29.0414, 16.428) (-28.9381, 16.3609) (-28.8341, 16.297) (-28.7279, 16.2346) knots 0 0 0 0 1 1 1 1
  spline S1448 degree 3 poles (-28.7279, 16.2346) (-28.5517, 16.1294) (-28.3853, 16.0111) (-28.2181, 15.8924) knots 0 0 0 0 1 1 1 1
  spline S1449 degree 3 poles (-28.2181, 15.8924) (-28.0992, 15.8083) (-27.9797, 15.7287) (-27.8538, 15.6555) knots 0 0 0 0 1 1 1 1
  spline S1450 degree 3 poles (-27.8538, 15.6555) (-27.663, 15.5435) (-27.4842, 15.4155) (-27.3037, 15.2878) knots 0 0 0 0 1 1 1 1
  spline S1451 degree 3 poles (-27.3037, 15.2878) (-27.0992, 15.1433) (-26.8958, 15.0016) (-26.6792, 14.8758) knots 0 0 0 0 1 1 1 1
  spline S1452 degree 3 poles (-26.6792, 14.8758) (-26.5668, 14.8084) (-26.4576, 14.737) (-26.348, 14.6652) knots 0 0 0 0 1 1 1 1
  spline S1453 degree 3 poles (-26.348, 14.6652) (-26.0462, 14.4677) (-25.7414, 14.2822) (-25.4233, 14.1117) knots 0 0 0 0 1 1 1 1
  spline S1454 degree 3 poles (-25.4233, 14.1117) (-25.3769, 14.0864) (-25.3305, 14.0611) (-25.2827, 14.035) knots 0 0 0 0 1 1 1 1
  spline S1455 degree 3 poles (-25.2827, 14.035) (-24.9335, 13.8467) (-24.5775, 13.6842) (-24.2074, 13.5412) knots 0 0 0 0 1 1 1 1
  spline S1456 degree 3 poles (-24.2074, 13.5412) (-24.1385, 13.5144) (-24.1385, 13.5144) (-24.0682, 13.4871) knots 0 0 0 0 1 1 1 1
  spline S1457 degree 3 poles (-24.0682, 13.4871) (-23.7687, 13.3792) (-23.4796, 13.3255) (-23.1659, 13.2844) knots 0 0 0 0 1 1 1 1
  spline S1458 degree 3 poles (-23.1659, 13.2844) (-22.3527, 13.1723) (-21.574, 12.8548) (-21.0051, 12.2471) knots 0 0 0 0 1 1 1 1
  spline S1459 degree 3 poles (-21.0051, 12.2471) (-20.8637, 12.295) (-20.7718, 12.3479) (-20.665, 12.4518) knots 0 0 0 0 1 1 1 1
  spline S1460 degree 3 poles (-20.665, 12.4518) (-20.6382, 12.4769) (-20.6114, 12.502) (-20.5838, 12.5278) knots 0 0 0 0 1 1 1 1
  spline S1461 degree 3 poles (-20.5838, 12.5278) (-20.5287, 12.5804) (-20.4739, 12.6333) (-20.4195, 12.6865) knots 0 0 0 0 1 1 1 1
  spline S1462 degree 3 poles (-20.4195, 12.6865) (-20.2269, 12.8654) (-20.0735, 12.9475) (-19.8079, 12.9539) knots 0 0 0 0 1 1 1 1
  spline S1463 degree 3 poles (-19.8079, 12.9539) (-19.5364, 12.9284) (-19.3024, 12.7893) (-19.0691, 12.6582) knots 0 0 0 0 1 1 1 1
  spline S1464 degree 3 poles (-19.0691, 12.6582) (-18.7642, 12.487) (-18.4593, 12.3893) (-18.123, 12.2987) knots 0 0 0 0 1 1 1 1
  spline S1465 degree 3 poles (-18.123, 12.2987) (-17.4825, 12.1239) (-16.8396, 11.8798) (-16.3889, 11.3675) knots 0 0 0 0 1 1 1 1
  spline S1466 degree 3 poles (-16.3889, 11.3675) (-16.3593, 11.2632) (-16.3593, 11.2632) (-16.3936, 11.1601) knots 0 0 0 0 1 1 1 1
  spline S1467 degree 3 poles (-16.3936, 11.1601) (-16.5099, 10.992) (-16.6468, 10.9076) (-16.8255, 10.8129) knots 0 0 0 0 1 1 1 1
  spline S1468 degree 3 poles (-16.8255, 10.8129) (-16.8702, 10.7887) (-16.9149, 10.7646) (-16.9609, 10.7398) knots 0 0 0 0 1 1 1 1
  spline S1469 degree 3 poles (-16.9609, 10.7398) (-17.3757, 10.5355) (-17.7803, 10.3989) (-18.2367, 10.3239) knots 0 0 0 0 1 1 1 1
  spline S1470 degree 3 poles (-18.2367, 10.3239) (-18.2875, 10.3154) (-18.3383, 10.3068) (-18.3906, 10.298) knots 0 0 0 0 1 1 1 1
  spline S1471 degree 3 poles (-18.3906, 10.298) (-18.8025, 10.2321) (-19.1989, 10.2055) (-19.6151, 10.2203) knots 0 0 0 0 1 1 1 1
  spline S1472 degree 3 poles (-19.6151, 10.2203) (-19.6506, 10.2213) (-19.6862, 10.2224) (-19.7228, 10.2234) knots 0 0 0 0 1 1 1 1
  spline S1473 degree 3 poles (-19.7228, 10.2234) (-19.9202, 10.2294) (-20.1173, 10.2373) (-20.3145, 10.2472) knots 0 0 0 0 1 1 1 1
  spline S1474 degree 3 poles (-20.3145, 10.2472) (-20.4956, 10.2559) (-20.676, 10.2594) (-20.8573, 10.2602) knots 0 0 0 0 1 1 1 1
  spline S1475 degree 3 poles (-20.8573, 10.2602) (-21.415, 10.2664) (-21.8382, 10.3149) (-22.3263, 10.5879) knots 0 0 0 0 1 1 1 1
  spline S1476 degree 3 poles (-22.3263, 10.5879) (-22.4869, 10.6744) (-22.6546, 10.7455) (-22.8213, 10.8193) knots 0 0 0 0 1 1 1 1
  spline S1477 degree 3 poles (-22.8213, 10.8193) (-23.1909, 10.9861) (-23.5588, 11.1563) (-23.9267, 11.3269) knots 0 0 0 0 1 1 1 1
  spline S1478 degree 3 poles (-23.9267, 11.3269) (-24.174, 11.4415) (-24.4216, 11.5554) (-24.6697, 11.668) knots 0 0 0 0 1 1 1 1
  spline S1479 degree 3 poles (-24.6697, 11.668) (-24.9764, 11.8073) (-25.2817, 11.9496) (-25.5868, 12.0922) knots 0 0 0 0 1 1 1 1
  spline S1480 degree 3 poles (-25.5868, 12.0922) (-25.846, 12.2132) (-26.106, 12.3325) (-26.3664, 12.4507) knots 0 0 0 0 1 1 1 1
  spline S1481 degree 3 poles (-26.3664, 12.4507) (-26.6082, 12.5607) (-26.8489, 12.6728) (-27.0896, 12.7852) knots 0 0 0 0 1 1 1 1
  spline S1482 degree 3 poles (-27.0896, 12.7852) (-27.1658, 12.8207) (-27.2421, 12.8562) (-27.3184, 12.8917) knots 0 0 0 0 1 1 1 1
  spline S1483 degree 3 poles (-27.3184, 12.8917) (-27.4598, 12.9575) (-27.6008, 13.0241) (-27.7415, 13.0914) knots 0 0 0 0 1 1 1 1
  spline S1484 degree 3 poles (-27.7415, 13.0914) (-28.2949, 13.3536) (-28.7646, 13.4941) (-29.3753, 13.3322) knots 0 0 0 0 1 1 1 1
  spline S1485 degree 3 poles (-29.3753, 13.3322) (-29.6719, 13.2111) (-30.0112, 13.0457) (-30.2331, 12.8092) knots 0 0 0 0 1 1 1 1
  spline S1486 degree 3 poles (-30.2331, 12.8092) (-30.2934, 12.6195) (-30.2695, 12.5032) (-30.1884, 12.3214) knots 0 0 0 0 1 1 1 1
  spline S1487 degree 3 poles (-30.1884, 12.3214) (-30.0953, 12.2239) (-30.0001, 12.1541) (-29.8877, 12.0801) knots 0 0 0 0 1 1 1 1
  spline S1488 degree 3 poles (-29.8877, 12.0801) (-29.625, 11.8873) (-29.2488, 11.604) (-29.1712, 11.2735) knots 0 0 0 0 1 1 1 1
  spline S1489 degree 3 poles (-29.1712, 11.2735) (-29.1678, 11.2378) (-29.1645, 11.2021) (-29.161, 11.1653) knots 0 0 0 0 1 1 1 1
  spline S1490 degree 3 poles (-29.161, 11.1653) (-29.1282, 10.946) (-29.066, 10.7998) (-28.902, 10.6481) knots 0 0 0 0 1 1 1 1
  spline S1491 degree 3 poles (-28.902, 10.6481) (-28.7551, 10.5576) (-28.6693, 10.5294) (-28.4971, 10.5336) knots 0 0 0 0 1 1 1 1
  spline S1492 degree 3 poles (-28.4971, 10.5336) (-28.202, 10.6279) (-27.9979, 10.8202) (-27.7799, 11.0333) knots 0 0 0 0 1 1 1 1
  spline S1493 degree 3 poles (-27.7799, 11.0333) (-27.6206, 11.1858) (-27.4902, 11.3072) (-27.2709, 11.3539) knots 0 0 0 0 1 1 1 1
  spline S1494 degree 3 poles (-27.2709, 11.3539) (-26.8205, 11.2921) (-26.4836, 10.9406) (-26.1558, 10.6521) knots 0 0 0 0 1 1 1 1
  spline S1495 degree 3 poles (-26.1558, 10.6521) (-25.9946, 10.512) (-25.8328, 10.3951) (-25.6469, 10.2901) knots 0 0 0 0 1 1 1 1
  spline S1496 degree 3 poles (-25.6469, 10.2901) (-25.2991, 10.0911) (-25.0783, 9.7733) (-24.9244, 9.408) knots 0 0 0 0 1 1 1 1
  spline S1497 degree 3 poles (-24.9244, 9.408) (-24.9664, 9.3867) (-25.0085, 9.3653) (-25.0518, 9.3433) knots 0 0 0 0 1 1 1 1
  spline S1498 degree 3 poles (-25.0518, 9.3433) (-25.1072, 9.3149) (-25.1627, 9.2865) (-25.2181, 9.2581) knots 0 0 0 0 1 1 1 1
  spline S1499 degree 3 poles (-25.2181, 9.2581) (-25.2458, 9.2441) (-25.2734, 9.2301) (-25.3019, 9.2156) knots 0 0 0 0 1 1 1 1
  spline S1500 degree 3 poles (-25.3019, 9.2156) (-25.5197, 9.1038) (-25.5197, 9.1038) (-25.6022, 9.0313) knots 0 0 0 0 1 1 1 1
  spline S1501 degree 3 poles (-25.6022, 9.0313) (-25.7255, 8.9564) (-25.8634, 8.9712) (-26.0037, 8.9699) knots 0 0 0 0 1 1 1 1
  spline S1502 degree 3 poles (-26.0037, 8.9699) (-26.3627, 8.9517) (-26.7198, 8.9256) (-27.0773, 8.8888) knots 0 0 0 0 1 1 1 1
  spline S1503 degree 3 poles (-27.0773, 8.8888) (-27.9448, 8.8003) (-28.7857, 8.7391) (-29.6521, 8.8842) knots 0 0 0 0 1 1 1 1